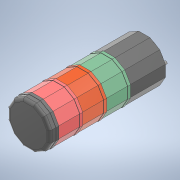
# Autodesk Inventor part: 503.024.01_Statuslampe
Saved by Autodesk Inventor 2021 (Build 250183000, 183)
## iProperties
Created: 2021-11-25
Part Number: 503.024.01_Statuslampe
Material: Generisch
Document SubType Name: Modeling
Designer: Sebastian Seewald
Density: 1 g/cm^3
Appearance: Vorgabe
Author: Sebastian Seewald
Autodesk Inventor part; units mm, degrees
ref_plane "YZ Plane" through (0, 0, 0) normal (1, 0, 0) x (0, 1, 0)
ref_plane "XZ Plane" through (0, 0, 0) normal (0, 1, 0) x (-1, 0, 0)
ref_plane "XY Plane" through (0, 0, 0) normal (0, 0, 1) x (1, 0, 0)
sketch "Skizze1" plane through (0, 0, 0) normal (0, 0, 1) x (1, 0, 0)
  line L0 (21.9615, -21.9615) -> (8.0385, -30)
  line L1 (8.0385, -30) -> (-8.0385, -30)
  line L2 (-8.0385, -30) -> (-21.9615, -21.9615)
  line L3 (-21.9615, -21.9615) -> (-30, -8.0385)
  line L4 (-30, -8.0385) -> (-30, 8.0385)
  line L5 (-30, 8.0385) -> (-21.9615, 21.9615)
  line L6 (-21.9615, 21.9615) -> (-8.0385, 30)
  line L7 (-8.0385, 30) -> (8.0385, 30)
  line L8 (8.0385, 30) -> (21.9615, 21.9615)
  line L9 (21.9615, 21.9615) -> (30, 8.0385)
  line L10 (30, 8.0385) -> (30, -8.0385)
  line L11 (30, -8.0385) -> (21.9615, -21.9615)
  line L12 (-42, 0) -> (42, 0) projected
  point P0 (0, 0)
  point P1 (0, 0)
  dimension "d0" = 60
  constraints: 24 end point, 1 coincident, 1 parallel, 25 other
  measures "d0" distance between parallel lines of L1 L7
extrude "Extrusion1" add sketch "Skizze1" along normal blind 50
sketch "Skizze2" plane through (0, 0, 50) normal (0, 0, 1) x (1, 0, 0)
  line L0 (21.9615, 21.9615) -> (8.0385, 30) projected
  line L1 (8.0385, 30) -> (-8.0385, 30) projected
  line L2 (-8.0385, 30) -> (-21.9615, 21.9615) projected
  line L3 (-21.9615, 21.9615) -> (-30, 8.0385) projected
  line L4 (-30, 8.0385) -> (-30, -8.0385) projected
  line L5 (-30, -8.0385) -> (-21.9615, -21.9615) projected
  line L6 (-21.9615, -21.9615) -> (-8.0385, -30) projected
  line L7 (-8.0385, -30) -> (8.0385, -30) projected
  line L8 (8.0385, -30) -> (21.9615, -21.9615) projected
  line L9 (21.9615, -21.9615) -> (30, -8.0385) projected
  line L10 (30, -8.0385) -> (30, 8.0385) projected
  line L11 (30, 8.0385) -> (21.9615, 21.9615) projected
  line L12 (-22.3275, 22.3275) -> (-8.1725, 30.5)
  line L13 (-8.1725, 30.5) -> (8.1725, 30.5)
  line L14 (8.1725, 30.5) -> (22.3275, 22.3275)
  line L15 (22.3275, 22.3275) -> (30.5, 8.1725)
  line L16 (30.5, 8.1725) -> (30.5, -8.1725)
  line L17 (30.5, -8.1725) -> (22.3275, -22.3275)
  line L18 (22.3275, -22.3275) -> (8.1725, -30.5)
  line L19 (8.1725, -30.5) -> (-8.1725, -30.5)
  line L20 (-8.1725, -30.5) -> (-22.3275, -22.3275)
  line L21 (-22.3275, -22.3275) -> (-30.5, -8.1725)
  line L22 (-30.5, -8.1725) -> (-30.5, 8.1725)
  line L23 (-30.5, 8.1725) -> (-22.3275, 22.3275)
  point P0 (0, 0)
  dimension "d3" = 0.5
  constraints: 24 end point, 11 other
  measures "d3" distance between parallel lines of L2 L12
extrude "Extrusion2" add sketch "Skizze2" along normal blind 4 contours L11 L10 L9 L8 L7 L6 L5 L4 L3 L2 L1 L0 | L12 L13 L14 L15 L16 L17 L18 L19 L20 L21 L22 L23
sketch "Skizze3" plane through (0, 0, 54) normal (0, 0, 1) x (1, 0, 0)
  line L0 (-30.5, 8.1725) -> (-30.5, -8.1725) projected
  line L1 (-30.5, -8.1725) -> (-22.3275, -22.3275) projected
  line L2 (-22.3275, -22.3275) -> (-8.1725, -30.5) projected
  line L3 (-8.1725, -30.5) -> (8.1725, -30.5) projected
  line L4 (8.1725, -30.5) -> (22.3275, -22.3275) projected
  line L5 (22.3275, -22.3275) -> (30.5, -8.1725) projected
  line L6 (30.5, -8.1725) -> (30.5, 8.1725) projected
  line L7 (30.5, 8.1725) -> (22.3275, 22.3275) projected
  line L8 (22.3275, 22.3275) -> (8.1725, 30.5) projected
  line L9 (8.1725, 30.5) -> (-8.1725, 30.5) projected
  line L10 (-8.1725, 30.5) -> (-22.3275, 22.3275) projected
  line L11 (-22.3275, 22.3275) -> (-30.5, 8.1725) projected
  line L12 (-30, -8.0385) -> (-30, 8.0385)
  line L13 (-30, 8.0385) -> (-21.9615, 21.9615)
  line L14 (-21.9615, 21.9615) -> (-8.0385, 30)
  line L15 (-8.0385, 30) -> (8.0385, 30)
  line L16 (8.0385, 30) -> (21.9615, 21.9615)
  line L17 (21.9615, 21.9615) -> (30, 8.0385)
  line L18 (30, 8.0385) -> (30, -8.0385)
  line L19 (30, -8.0385) -> (21.9615, -21.9615)
  line L20 (21.9615, -21.9615) -> (8.0385, -30)
  line L21 (8.0385, -30) -> (-8.0385, -30)
  line L22 (-8.0385, -30) -> (-21.9615, -21.9615)
  line L23 (-21.9615, -21.9615) -> (-30, -8.0385)
  point P0 (0, 0)
  dimension "d6" = 0.5
  constraints: 24 end point, 11 other
  measures "d6" distance between parallel lines of L0 L12
extrude "Extrusion3" add sketch "Skizze3" along normal blind 30 contours L12 L13 L14 L15 L16 L17 L18 L19 L20 L21 L22 L23
sketch "Skizze4" plane through (0, 0, 84) normal (0, 0, 1) x (1, 0, 0)
  line L0 (-21.9615, -21.9615) -> (-8.0385, -30) projected
  line L1 (-8.0385, -30) -> (8.0385, -30) projected
  line L2 (8.0385, -30) -> (21.9615, -21.9615) projected
  line L3 (21.9615, -21.9615) -> (30, -8.0385) projected
  line L4 (30, -8.0385) -> (30, 8.0385) projected
  line L5 (30, 8.0385) -> (21.9615, 21.9615) projected
  line L6 (21.9615, 21.9615) -> (8.0385, 30) projected
  line L7 (8.0385, 30) -> (-8.0385, 30) projected
  line L8 (-8.0385, 30) -> (-21.9615, 21.9615) projected
  line L9 (-21.9615, 21.9615) -> (-30, 8.0385) projected
  line L10 (-30, 8.0385) -> (-30, -8.0385) projected
  line L11 (-30, -8.0385) -> (-21.9615, -21.9615) projected
  line L12 (-30.5, -8.1725) -> (-30.5, 8.1725)
  line L13 (-30.5, 8.1725) -> (-22.3275, 22.3275)
  line L14 (-22.3275, 22.3275) -> (-8.1725, 30.5)
  line L15 (-8.1725, 30.5) -> (8.1725, 30.5)
  line L16 (8.1725, 30.5) -> (22.3275, 22.3275)
  line L17 (22.3275, 22.3275) -> (30.5, 8.1725)
  line L18 (30.5, 8.1725) -> (30.5, -8.1725)
  line L19 (30.5, -8.1725) -> (22.3275, -22.3275)
  line L20 (22.3275, -22.3275) -> (8.1725, -30.5)
  line L21 (8.1725, -30.5) -> (-8.1725, -30.5)
  line L22 (-8.1725, -30.5) -> (-22.3275, -22.3275)
  line L23 (-22.3275, -22.3275) -> (-30.5, -8.1725)
  point P0 (0, 0)
  dimension "d9" = 0.5
  constraints: 24 end point, 11 other
  measures "d9" distance between parallel lines of L10 L12
extrude "Extrusion4" add sketch "Skizze4" along normal blind 4 contours L11 L10 L9 L8 L7 L6 L5 L4 L3 L2 L1 L0 | L12 L13 L14 L15 L16 L17 L18 L19 L20 L21 L22 L23
sketch "Skizze5" plane through (0, 0, 88) normal (0, 0, 1) x (1, 0, 0)
  line L0 (-22.3275, -22.3275) -> (-8.1725, -30.5) projected
  line L1 (-8.1725, -30.5) -> (8.1725, -30.5) projected
  line L2 (8.1725, -30.5) -> (22.3275, -22.3275) projected
  line L3 (22.3275, -22.3275) -> (30.5, -8.1725) projected
  line L4 (30.5, -8.1725) -> (30.5, 8.1725) projected
  line L5 (30.5, 8.1725) -> (22.3275, 22.3275) projected
  line L6 (22.3275, 22.3275) -> (8.1725, 30.5) projected
  line L7 (8.1725, 30.5) -> (-8.1725, 30.5) projected
  line L8 (-8.1725, 30.5) -> (-22.3275, 22.3275) projected
  line L9 (-22.3275, 22.3275) -> (-30.5, 8.1725) projected
  line L10 (-30.5, 8.1725) -> (-30.5, -8.1725) projected
  line L11 (-30.5, -8.1725) -> (-22.3275, -22.3275) projected
  line L12 (-30, -8.0385) -> (-30, 8.0385)
  line L13 (-30, 8.0385) -> (-21.9615, 21.9615)
  line L14 (-21.9615, 21.9615) -> (-8.0385, 30)
  line L15 (-8.0385, 30) -> (8.0385, 30)
  line L16 (8.0385, 30) -> (21.9615, 21.9615)
  line L17 (21.9615, 21.9615) -> (30, 8.0385)
  line L18 (30, 8.0385) -> (30, -8.0385)
  line L19 (30, -8.0385) -> (21.9615, -21.9615)
  line L20 (21.9615, -21.9615) -> (8.0385, -30)
  line L21 (8.0385, -30) -> (-8.0385, -30)
  line L22 (-8.0385, -30) -> (-21.9615, -21.9615)
  line L23 (-21.9615, -21.9615) -> (-30, -8.0385)
  point P0 (0, 0)
  dimension "d12" = 0.5
  constraints: 24 end point, 11 other
  measures "d12" distance between parallel lines of L10 L12
extrude "Extrusion5" add sketch "Skizze5" along normal blind 30 contours L12 L13 L14 L15 L16 L17 L18 L19 L20 L21 L22 L23
sketch "Skizze6" plane through (0, 0, 118) normal (0, 0, 1) x (1, 0, 0)
  line L0 (-21.9615, -21.9615) -> (-8.0385, -30) projected
  line L1 (-8.0385, -30) -> (8.0385, -30) projected
  line L2 (8.0385, -30) -> (21.9615, -21.9615) projected
  line L3 (21.9615, -21.9615) -> (30, -8.0385) projected
  line L4 (30, -8.0385) -> (30, 8.0385) projected
  line L5 (30, 8.0385) -> (21.9615, 21.9615) projected
  line L6 (21.9615, 21.9615) -> (8.0385, 30) projected
  line L7 (8.0385, 30) -> (-8.0385, 30) projected
  line L8 (-8.0385, 30) -> (-21.9615, 21.9615) projected
  line L9 (-21.9615, 21.9615) -> (-30, 8.0385) projected
  line L10 (-30, 8.0385) -> (-30, -8.0385) projected
  line L11 (-30, -8.0385) -> (-21.9615, -21.9615) projected
  line L12 (-22.3275, -22.3275) -> (-8.1725, -30.5)
  line L13 (-8.1725, -30.5) -> (8.1725, -30.5)
  line L14 (8.1725, -30.5) -> (22.3275, -22.3275)
  line L15 (22.3275, -22.3275) -> (30.5, -8.1725)
  line L16 (30.5, -8.1725) -> (30.5, 8.1725)
  line L17 (30.5, 8.1725) -> (22.3275, 22.3275)
  line L18 (22.3275, 22.3275) -> (8.1725, 30.5)
  line L19 (8.1725, 30.5) -> (-8.1725, 30.5)
  line L20 (-8.1725, 30.5) -> (-22.3275, 22.3275)
  line L21 (-22.3275, 22.3275) -> (-30.5, 8.1725)
  line L22 (-30.5, 8.1725) -> (-30.5, -8.1725)
  line L23 (-30.5, -8.1725) -> (-22.3275, -22.3275)
  point P0 (0, 0)
  dimension "d15" = 0.5
  constraints: 24 end point, 11 other
  measures "d15" distance between parallel lines of L10 L22
extrude "Extrusion6" add sketch "Skizze6" along normal blind 4 contours L11 L10 L9 L8 L7 L6 L5 L4 L3 L2 L1 L0 | L23 L22 L21 L20 L19 L18 L17 L16 L15 L14 L13 L12
sketch "Skizze7" plane through (0, 0, 122) normal (0, 0, 1) x (1, 0, 0)
  line L0 (-8.1725, -30.5) -> (8.1725, -30.5) projected
  line L1 (8.1725, -30.5) -> (22.3275, -22.3275) projected
  line L2 (22.3275, -22.3275) -> (30.5, -8.1725) projected
  line L3 (30.5, -8.1725) -> (30.5, 8.1725) projected
  line L4 (30.5, 8.1725) -> (22.3275, 22.3275) projected
  line L5 (22.3275, 22.3275) -> (8.1725, 30.5) projected
  line L6 (8.1725, 30.5) -> (-8.1725, 30.5) projected
  line L7 (-8.1725, 30.5) -> (-22.3275, 22.3275) projected
  line L8 (-22.3275, 22.3275) -> (-30.5, 8.1725) projected
  line L9 (-30.5, 8.1725) -> (-30.5, -8.1725) projected
  line L10 (-30.5, -8.1725) -> (-22.3275, -22.3275) projected
  line L11 (-22.3275, -22.3275) -> (-8.1725, -30.5) projected
  line L12 (-21.9615, -21.9615) -> (-30, -8.0385)
  line L13 (-30, -8.0385) -> (-30, 8.0385)
  line L14 (-30, 8.0385) -> (-21.9615, 21.9615)
  line L15 (-21.9615, 21.9615) -> (-8.0385, 30)
  line L16 (-8.0385, 30) -> (8.0385, 30)
  line L17 (8.0385, 30) -> (21.9615, 21.9615)
  line L18 (21.9615, 21.9615) -> (30, 8.0385)
  line L19 (30, 8.0385) -> (30, -8.0385)
  line L20 (30, -8.0385) -> (21.9615, -21.9615)
  line L21 (21.9615, -21.9615) -> (8.0385, -30)
  line L22 (8.0385, -30) -> (-8.0385, -30)
  line L23 (-8.0385, -30) -> (-21.9615, -21.9615)
  point P0 (0, 0)
  dimension "d18" = 0.5
  constraints: 24 end point, 11 other
  measures "d18" distance between parallel lines of L9 L13
extrude "Extrusion7" add sketch "Skizze7" along normal blind 30 contours L12 L13 L14 L15 L16 L17 L18 L19 L20 L21 L22 L23
sketch "Skizze8" plane through (0, 0, 152) normal (0, 0, 1) x (1, 0, 0)
  line L0 (-8.0385, -30) -> (8.0385, -30) projected
  line L1 (8.0385, -30) -> (21.9615, -21.9615) projected
  line L2 (21.9615, -21.9615) -> (30, -8.0385) projected
  line L3 (30, -8.0385) -> (30, 8.0385) projected
  line L4 (30, 8.0385) -> (21.9615, 21.9615) projected
  line L5 (21.9615, 21.9615) -> (8.0385, 30) projected
  line L6 (8.0385, 30) -> (-8.0385, 30) projected
  line L7 (-8.0385, 30) -> (-21.9615, 21.9615) projected
  line L8 (-21.9615, 21.9615) -> (-30, 8.0385) projected
  line L9 (-30, 8.0385) -> (-30, -8.0385) projected
  line L10 (-30, -8.0385) -> (-21.9615, -21.9615) projected
  line L11 (-21.9615, -21.9615) -> (-8.0385, -30) projected
  line L12 (-30.5, -8.1725) -> (-30.5, 8.1725)
  line L13 (-30.5, 8.1725) -> (-22.3275, 22.3275)
  line L14 (-22.3275, 22.3275) -> (-8.1725, 30.5)
  line L15 (-8.1725, 30.5) -> (8.1725, 30.5)
  line L16 (8.1725, 30.5) -> (22.3275, 22.3275)
  line L17 (22.3275, 22.3275) -> (30.5, 8.1725)
  line L18 (30.5, 8.1725) -> (30.5, -8.1725)
  line L19 (30.5, -8.1725) -> (22.3275, -22.3275)
  line L20 (22.3275, -22.3275) -> (8.1725, -30.5)
  line L21 (8.1725, -30.5) -> (-8.1725, -30.5)
  line L22 (-8.1725, -30.5) -> (-22.3275, -22.3275)
  line L23 (-22.3275, -22.3275) -> (-30.5, -8.1725)
  point P0 (0, 0)
  dimension "d21" = 0.5
  constraints: 24 end point, 11 other
  measures "d21" distance between parallel lines of L9 L12
extrude "Extrusion8" add sketch "Skizze8" along normal blind 4 contours L11 L10 L9 L8 L7 L6 L5 L4 L3 L2 L1 L0 | L12 L13 L14 L15 L16 L17 L18 L19 L20 L21 L22 L23
sketch "Skizze9" plane through (0, 0, 156) normal (0, 0, 1) x (1, 0, 0)
  line L0 (-22.3275, -22.3275) -> (-8.1725, -30.5) projected
  line L1 (-8.1725, -30.5) -> (8.1725, -30.5) projected
  line L2 (8.1725, -30.5) -> (22.3275, -22.3275) projected
  line L3 (22.3275, -22.3275) -> (30.5, -8.1725) projected
  line L4 (30.5, -8.1725) -> (30.5, 8.1725) projected
  line L5 (30.5, 8.1725) -> (22.3275, 22.3275) projected
  line L6 (22.3275, 22.3275) -> (8.1725, 30.5) projected
  line L7 (8.1725, 30.5) -> (-8.1725, 30.5) projected
  line L8 (-8.1725, 30.5) -> (-22.3275, 22.3275) projected
  line L9 (-22.3275, 22.3275) -> (-30.5, 8.1725) projected
  line L10 (-30.5, 8.1725) -> (-30.5, -8.1725) projected
  line L11 (-30.5, -8.1725) -> (-22.3275, -22.3275) projected
  line L12 (-30, -8.0385) -> (-30, 8.0385)
  line L13 (-30, 8.0385) -> (-21.9615, 21.9615)
  line L14 (-21.9615, 21.9615) -> (-8.0385, 30)
  line L15 (-8.0385, 30) -> (8.0385, 30)
  line L16 (8.0385, 30) -> (21.9615, 21.9615)
  line L17 (21.9615, 21.9615) -> (30, 8.0385)
  line L18 (30, 8.0385) -> (30, -8.0385)
  line L19 (30, -8.0385) -> (21.9615, -21.9615)
  line L20 (21.9615, -21.9615) -> (8.0385, -30)
  line L21 (8.0385, -30) -> (-8.0385, -30)
  line L22 (-8.0385, -30) -> (-21.9615, -21.9615)
  line L23 (-21.9615, -21.9615) -> (-30, -8.0385)
  point P0 (0, 0)
  dimension "d24" = 0.5
  constraints: 24 end point, 11 other
  measures "d24" distance between parallel lines of L10 L12
extrude "Extrusion9" add sketch "Skizze9" along normal blind 9 contours L12 L13 L14 L15 L16 L17 L18 L19 L20 L21 L22 L23
fillet "Rundung1" radius 4 12 edges at (25.9808, -15, 165) (30, 0, 165) (25.9808, 15, 165) (15, 25.9808, 165) (0, 30, 165) (-15, 25.9808, 165) (-25.9808, 15, 165) (-30, 0, 165) (-25.9808, -15, 165) (-15, -25.9808, 165) (0, -30, 165) (15, -25.9808, 165)
sketch "Skizze10" plane through (0, 0, 0) normal (0, 0, -1) x (-1, 0, 0)
  point P0 (0, 0)
  point P1 (-20, 0)
  point P2 (20, 0)
  dimension "d35" = 20
  dimension "d36" = 20
  constraints: 2 horizontal alignment
  measures "d35" distance of point (0, 0) point (-20, 0)
  measures "d36" distance of point (0, 0) point (20, 0)
hole "Bohrung1" at (20, 0, 0) at (-20, 0, 0) direction (0, 0, 1) diameter 4.917 depth 17.1 thread size "M6x1" class "6H" standard "ISO Metric profile"
sketch "Skizze11" plane through (0, 0, 0) normal (0, 0, -1) x (-1, 0, 0)
  circle A0 centre (0, 0) radius 12.5
  dimension "d37" = 25
  constraints: 1 centre point, 1 coincident
  measures "d37" diameter of A0
extrude "Extrusion10" cut sketch "Skizze11" against normal blind 15
sketch "Skizze12" plane through (0, 0, 15) normal (0, 0, -1) x (-1, 0, 0)
  circle A0 centre (2, 0) radius 1.5
  circle A1 centre (-2, 0) radius 1.5
  circle A2 centre (0, 3) radius 1.5
  circle A3 centre (0, -3) radius 1.5
  point P0 (0, 0)
  dimension "d40" = 3
  dimension "d41" = 3
  dimension "d42" = 2
  dimension "d43" = 2
  dimension "d50" = 3
  dimension "d51" = 3
  dimension "d52" = 3
  dimension "d53" = 3
  constraints: 4 centre point, 2 horizontal alignment, 2 vertical alignment
  measures "d40" diameter of A1
  measures "d41" diameter of A0
  measures "d42" distance of point (0, 0) A1.centre
  measures "d43" distance of point (0, 0) A0.centre
  measures "d50" diameter of A2
  measures "d51" diameter of A3
  measures "d52" distance of point (0, 0) A3.centre
  measures "d53" distance of point (0, 0) A2.centre
extrude "Extrusion11" add sketch "Skizze12" along normal blind 25
sketch "Skizze13" plane through (0, 0, 15) normal (0, 0, -1) x (-1, 0, 0)
  circle A0 centre (0, 0) radius 7.5
  circle A1 centre (0, 0) radius 6.5
  dimension "d46" = 15
  dimension "d47" = 13
  constraints: 2 centre point, 2 coincident
  measures "d46" diameter of A0
  measures "d47" diameter of A1
extrude "Extrusion12" add sketch "Skizze13" along normal blind 15
sketch "Skizze14" plane through (0, 0, 0) normal (0, 0, -1) x (-1, 0, 0)
  circle A0 centre (0, 0) radius 29.5
  circle A1 centre (0, 0) radius 13
  circle A2 centre (-20, 0) radius 2.4585 projected
  circle A3 centre (20, 0) radius 2.4585 projected
  dimension "d54" = 26
  dimension "d55" = 59
  constraints: 2 centre point, 2 coincident
  measures "d54" diameter of A1
  measures "d55" diameter of A0
extrude "Extrusion13" add sketch "Skizze14" along normal blind 0.5
sketch "Skizze15" plane through (0, 0, -0.5) normal (0, 0, -1) x (-1, 0, 0)
  circle A0 centre (-20, 0) radius 2.4585 projected
  circle A1 centre (20, 0) radius 2.4585 projected
  circle A2 centre (-20, 0) radius 2
  circle A3 centre (20, 0) radius 2
  point P0 (0, 0)
  dimension "d62" = 4
  dimension "d63" = 4
  constraints: 2 centre point
  measures "d62" diameter of A2
  measures "d63" diameter of A3
extrude "Extrusion14" add sketch "Skizze15" along normal blind 10 and the other way blind 20 contours A2 | A3
thread "Gewinde1" size "M4x0.5" class "6g" standard "ANSI Metric M Profile" length 50
thread "Gewinde2" size "M4x0.5" class "6g" standard "ANSI Metric M Profile" length 50
